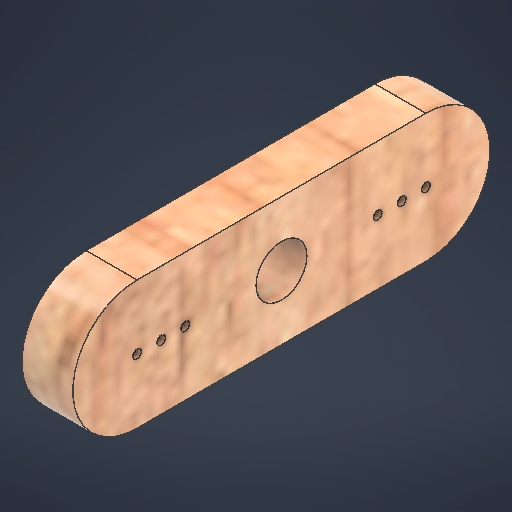
# Autodesk Inventor part: Spacer Skiba
Saved by Autodesk Inventor 2027.1 (Build 311270010, 270A)
## iProperties
Created: 2024-10-30
Part Number: Spacer Skiba
Material: Generic
Document SubType Name: Modeling
Designer: 239tr
Density: 1 g/cm^3
Appearance: Birch - Natural Polished
Mass: 4.69704 g
Surface Area: 25.1411 cm^2
Volume: 4.69704 cm^3
Author: 239tr
Autodesk Inventor part; units mm, degrees
ref_plane "YZ Plane" through (0, 0, 0) normal (1, 0, 0) x (0, 1, 0)
ref_plane "XZ Plane" through (0, 0, 0) normal (0, 1, 0) x (-1, 0, 0)
ref_plane "XY Plane" through (0, 0, 0) normal (0, 0, 1) x (1, 0, 0)
sketch "Block1" plane through (0, 0, 0) normal (0, 0, 1) x (1, 0, 0)
  circle A0 centre (-34.5082, -40.3774) radius 0.55
  circle A1 centre (-31.5082, -40.3774) radius 0.55
  circle A2 centre (-28.5082, -40.3774) radius 0.55
  point P0 (-31.5082, -40.3774)
  dimension "d7" = 1.1
  dimension "d8" = 1.1
  dimension "d9" = 1.1
  measures "d7" diameter of A0
  measures "d8" diameter of A1
  measures "d9" diameter of A2
sketch "Sketch1" plane through (0, 0, 0) normal (1, 0, 0) x (0, 1, 0)
  circle A0 centre (0, 0) radius 3.175
  line L0 (8, 0) -> (8, -60)
  line L1 (-8, 0) -> (-8, -60)
  arc A1 (-8, -60) -> (8, -60) centre (0, -60) ccw
  circle A2 centre (0, -60) radius 3.175
  line L2 (0, -105.9654) -> (0, 47.9942) construction
  line L3 (8, 0) -> (-8, 0) construction
  line L4 (8, 0) -> (8, 18)
  line L5 (-8, 0) -> (-8, 18)
  arc A3 (8, 18) -> (-8, 18) centre (0, 18) ccw
  line L6 (-36, 0) -> (58.5, 0) construction
  line L7 (0, -45) -> (-22.5, -83.9711)
  line L8 (0, -45) -> (45, -45) construction
  line L9 (-22.5, -83.9711) -> (-22.5, -45)
  line L10 (-22.5, -45) -> (0, -45)
  line L11 (-22.5, -45) -> (-8, -30)
  circle A4 centre (0, -18) radius 8
  circle A5 centre (0, -12) radius 0.55
  circle A6 centre (0, -15) radius 0.55
  circle A7 centre (0, -18) radius 0.55
  circle A8 centre (0, 12) radius 0.55
  circle A9 centre (0, 15) radius 0.55
  circle A10 centre (0, 18) radius 0.55
  point P0 (0, 0)
  point P1 (-8, -58.8564)
  point P2 (-8, -18)
  point P3 (8, -18)
  dimension "d0" = 6.35
  dimension "d2" = 16
  dimension "d4" = 6.35
  dimension "d11" = 12
  dimension "d12" = 60
  dimension "d13" = 45
  dimension "d14" = 120
  dimension "d15" = 45
  constraints: 20 end point, 9 vertical, 5 centre point, 5 tangent, 4 point on circle, 2 coincident, 2 horizontal, 2 midpoint, 1 collinear, 1 equal length, 1 point on line, 2 other
  measures "d0" diameter of A0
  measures "d2" diameter of A1
  measures "d4" diameter of A2
  measures "d12" distance of A1.centre A0.centre
  measures "d13" distance of L7.start L7.end
  measures "d14" angle of L7 L8
  measures "d15" distance of point (0, 0) L7.start
extrude "Extrusion2" add sketch "Sketch1" along normal blind 6.35 contours L0 A4 L1 L5 A3 L4 | A4
equation "\"d7\" = d9"
equation "\"d8\" = d9"
body "Solid2"
